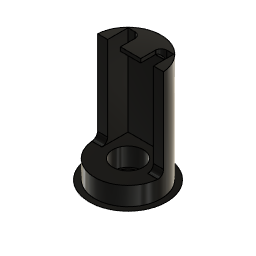
TDS_stake_pipe_connector v1 (Autodesk Fusion 360 design; units mm, degrees)
Autodesk Fusion 360 part; units mm, degrees
sketch "Sketch1" plane through (0, 0, 0) normal (0, 1, 0) x (1, 0, 0)
  line L0 (6.325, 0) -> (6.325, -15)
  line L1 (6.325, 0) -> (8.325, 0)
  line L2 (8.325, -15) -> (12.025, -15)
  line L3 (12.025, -15) -> (12.025, -29.5)
  line L4 (12.025, -29.5) -> (26, -29.5)
  line L5 (26, -29.5) -> (26, -15)
  line L6 (26, -15) -> (30.3, -15)
  line L7 (6.325, -15) -> (2.8, -15)
  line L8 (2.8, -15) -> (2.8, -16.5)
  line L9 (2.8, -16.5) -> (8.325, -16.5)
  line L10 (8.325, -16.5) -> (8.325, -15)
  line L11 (8.325, 0) -> (30.3, -15)
  dimension "d1" = 6.325
  dimension "d3" = 2
  dimension "d4" = 5.7
  dimension "d5" = 14.5
  dimension "d6" = 13.975
  dimension "d7" = 4.3
  dimension "d8" = 3.525
  dimension "d9" = 1.5
  dimension "d10" = 5.525
  constraint horizontal L1
  constraint perpendicular L0 L2
  constraint perpendicular L2 L3
  constraint perpendicular L3 L4
  constraint perpendicular L4 L5
  constraint perpendicular L5 L6
  constraint perpendicular L0 L7
  constraint perpendicular L7 L8
  constraint perpendicular L0 L9
  constraint perpendicular L2 L10
  measures "d1" distance of origin L0.start
  measures "d3" distance of L0.start L1.end
  measures "d4" distance of L0.end L2.end
  measures "d5" distance of L2.end L3.end
  measures "d6" distance of L3.end L4.end
  measures "d7" distance of L5.end L6.end
  measures "d8" distance of L0.end L7.end
  measures "d9" distance of L7.end L8.end
  measures "d10" distance of L8.end L9.end
revolve "Revolve1" add sketch "Sketch1" angle 360 about axis through (0, 0, 1.75) along (0, 0, 1)
ref_plane "WorkPlane1" through (8.325, 0, 15.2437) normal (1, 0, 0) x (0, -1, 0)
sketch "Sketch2" plane through (8.325, 0, 15.2437) normal (1, 0, 0) x (0, 1, 0)
  circle A0 centre (0, 0.5) radius 0.5
extrude "Extrude1" cut sketch "Sketch2" against normal blind 8
sketch "Sketch3" plane through (0, 0, 15) normal (0, 0, -1) x (1, 0, 0)
  circle A0 centre (0, 0) radius 2.8
  circle A1 centre (0, 0) radius 6.325
  line L0 (0, 2.8) -> (-5.6715, 2.8)
  line L1 (0, -2.8) -> (-5.6715, -2.8)
  arc A2 (-5.6715, 2.8) -> (-5.6715, -2.8) centre (0, 0) ccw
  constraint coincident A0.centre A1.centre
  constraint coincident A0 L0.start
  constraint coincident A1 L0.end
  constraint tangent A0 L0
  constraint coincident A0 L1.start
  constraint tangent A0 L1
extrude "Extrude2" cut sketch "Sketch3" against normal blind 114 contours A0 A1 L0 L1 A2
sketch "Sketch4" plane through (0, 0, 29.5) normal (0, 0, 1) x (-1, 0, 0)
  circle A0 centre (0, 0) radius 26
  circle A1 centre (0, 0) radius 12.025
  line L0 (0, -18) -> (-18, -18)
  line L1 (0, -18) -> (18, -18)
  line L2 (-18, -18) -> (-18, -2)
  line L3 (-18, -2) -> (-25.923, -2)
  line L4 (18, -18) -> (18, -2)
  line L5 (18, -2) -> (25.923, -2)
  arc A2 (-25.923, -2) -> (25.923, -2) centre (0, 0) ccw
  dimension "d17" = 18
  dimension "d18" = 18
  constraint horizontal L0
  constraint parallel L0 L1
  constraint perpendicular L0 L2
  constraint coincident A0 L3.end
  constraint perpendicular L2 L3
  constraint perpendicular L1 L4
  constraint coincident A0 L5.end
  constraint perpendicular L4 L5
  constraint coincident A0.centre A1.centre
  measures "d17" distance of L0.start L0.end
  measures "d18" distance of L0.start L1.end
extrude "Extrude3" add sketch "Sketch4" along normal blind 68 contours A0 L0 L1 L2 L3 L4 L5 A2
sketch "Sketch5" plane through (0, 0, 97.5) normal (0, 0, 1) x (-1, 0, 0)
  line L0 (18, -18) -> (-18, -18)
  line L1 (-18, -18) -> (-18, -2)
  line L2 (-18, -2) -> (-25.923, -2)
  arc A0 (-25.923, -2) -> (25.923, -2) centre (0, 0) ccw
  line L3 (25.923, -2) -> (18, -2)
  line L4 (18, -2) -> (18, -18)
  line L5 (0, -18) -> (-8, -18)
  line L6 (0, -18) -> (8, -18)
  line L7 (8, -18) -> (8, -2)
  line L8 (8, -2) -> (-8, -2)
  line L9 (-8, -2) -> (-8, -18)
  dimension "d21" = 8
  dimension "d22" = 8
  constraint midpoint L0 L5.start
  constraint perpendicular L4 L5
  constraint parallel L0 L6
  constraint perpendicular L3 L7
  constraint perpendicular L7 L8
  constraint perpendicular L5 L9
  measures "d21" distance of L5.start L5.end
  measures "d22" distance of L5.start L6.end
extrude "Extrude4" add sketch "Sketch5" along normal blind 3
fillet "Fillet1" radius 4.5 1 edges at (-8, 18, 99)
fillet "Fillet2" radius 4.5 1 edges at (8, 18, 99)
fillet "Fillet3" radius 4.5 1 edges at (0, 18, 97.5)
fillet "Fillet4" radius 4.5 2 edges at (21.9615, 2, 29.5) (-21.9615, 2, 29.5)
